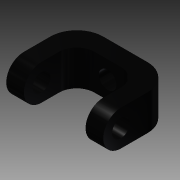
# Autodesk Inventor part: EE_base_connection
Saved by Autodesk Inventor 2015 (Build 190159000, 159)
## iProperties
Created: 2017-04-04
Part Number: EE_base_connection
Material: Acetal Resin, Black
Document SubType Name: Modeling
Designer: Guy
Density: 1.425 g/cm^3
Appearance: Smooth - Black
Author: Guy
Autodesk Inventor part; units mm, degrees
ref_plane "YZ Plane" through (0, 0, 0) normal (1, 0, 0) x (0, 1, 0)
ref_plane "XZ Plane" through (0, 0, 0) normal (0, 1, 0) x (-1, 0, 0)
ref_plane "XY Plane" through (0, 0, 0) normal (0, 0, 1) x (1, 0, 0)
sketch "Sketch1" plane through (0, 0, 0) normal (0, 0, 1) x (1, 0, 0)
  line L0 (0, 0) -> (10, 0)
  line L1 (10, 0) -> (10, 30)
  line L2 (10, 30) -> (45, 30)
  line L3 (45, 30) -> (45, 0)
  line L4 (45, 0) -> (55, 0)
  line L5 (55, 0) -> (55, 40)
  line L6 (55, 40) -> (0, 40)
  line L7 (0, 40) -> (0, 0)
  dimension "d0" = 10
  dimension "d1" = 35
  dimension "d2" = 10
  dimension "d3" = 40
  dimension "d4" = 10
  constraints: 16 end point, 6 perpendicular, 2 point on line, 1 horizontal
  measures "d0" distance of L0.start L0.end
  measures "d1" distance between parallel lines of L3 L1
  measures "d2" distance of L3.end L4.end
  measures "d3" distance of L6.end L0.start
  measures "d4" distance between parallel lines of L6 L2
extrude "Extrusion1" add sketch "Sketch1" along normal blind 20
sketch "Sketch2" plane through (55, 0, 0) normal (1, 0, 0) x (0, 0, -1)
  circle A0 centre (-10, 10) radius 5
  line L0 (0, 0) -> (0, 40) projected
  line L1 (0, 0) -> (0, 40) projected
  line L2 (0, 40) -> (-20, 40) projected
  line L3 (-20, 0) -> (-20, 40) projected
  line L4 (0, 0) -> (-20, 0) projected
  dimension "d7" = 10
  dimension "d8" = 10
  dimension "d9" = 20
  dimension "d10" = 10
  constraints: 1 centre point
  measures "d7" diameter of A0
  measures "d8" distance from line of L0 A0.centre
  measures "d9" distance of L1.start L3.start
  measures "d10" distance from line of L4 A0.centre
extrude "Extrusion2" cut sketch "Sketch2" against normal through all contours A0
sketch "Sketch3" plane through (0, 40, 0) normal (0, 1, 0) x (1, 0, 0)
  line L0 (55, 0) -> (0, 0) projected
  line L1 (0, 0) -> (0, -20) projected
  line L2 (55, -20) -> (0, -20) projected
  line L3 (55, 0) -> (55, -20) projected
  circle A0 centre (27.5, -10) radius 5
  point P0 (0, 0)
  dimension "d13" = 55
  dimension "d14" = 10
  dimension "d15" = 27.5
  dimension "d16" = 20
  dimension "d17" = 10
  constraints: 1 centre point
  measures "d13" distance of L2.start L1.end
  measures "d14" diameter of A0
  measures "d15" distance from line of A0.centre L1
  measures "d16" distance of L0.end L1.end
  measures "d17" distance from line of L2 A0.centre
extrude "Extrusion3" cut sketch "Sketch3" against normal up to next contours A0
fillet "Fillet1" radius 10 4 edges at (5, 0, 20) (5, 0, 0) (50, 0, 20) (50, 0, 0)
fillet "Fillet2" radius 10 2 edges at (10, 30, 10) (45, 30, 10)
fillet "Fillet4" radius 15 2 edges at (0, 40, 10) (55, 40, 10)
equation "\"d8\" = 0.5 * d9"
equation "\"d15\" = 0.5 * d13"
equation "\"d17\" = 0.5 * d16"
body "Solid1"
